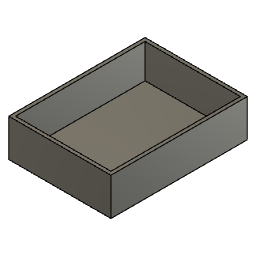
Box (Autodesk Fusion 360 design; units mm, degrees)
Autodesk Fusion 360 part; units mm, degrees
sketch "Sketch1" plane through (0, 0, 0) normal (0, 1, 0) x (1, 0, 0)
  line L0 (0, 0) -> (300, 0)
  line L1 (300, 0) -> (300, 400)
  line L2 (300, 400) -> (0, 400)
  line L3 (0, 400) -> (0, 0)
  line L4 (0, 0) -> (10, 0)
  line L5 (0, 0) -> (9.8603, 0)
  line L6 (0, 10) -> (0, 0)
  line L7 (9.8603, 10) -> (289.8603, 10)
  line L8 (289.8603, 10) -> (289.8603, 390)
  line L9 (289.8603, 390) -> (9.8603, 390)
  line L10 (9.8603, 390) -> (9.8603, 10)
  constraint horizontal L0
  constraint vertical L1
  constraint horizontal L2
  constraint vertical L3
  constraint coincident L0.start L3.end
  constraint perpendicular L3 L4
  constraint horizontal L5
  constraint vertical L6
  constraint horizontal L7
  constraint vertical L8
  constraint horizontal L9
  constraint vertical L10
extrude "Extrude1" add sketch "Sketch1" along normal blind 10 contours L0 L1 L2 L3 L4 L5 L6 | L7 L8 L9 L10
sketch "Sketch2" plane through (0, 10, 0) normal (0, 1, 0) x (-1, 0, 0)
  line L0 (0, -400) -> (0, 0)
  line L1 (0, 0) -> (-300, 0)
  line L2 (-300, 0) -> (-300, -400)
  line L3 (-300, -400) -> (0, -400)
  line L4 (0, 0) -> (-10, 0)
  line L5 (0, -10) -> (0, 0)
  line L6 (-10, -10) -> (-290, -10)
  line L7 (-290, -10) -> (-290, -390)
  line L8 (-290, -390) -> (-10, -390)
  line L9 (-10, -390) -> (-10, -10)
  line L10 (0, 0) -> (-300, 0)
  line L11 (-300, 0) -> (-300, -400)
  line L12 (-300, -400) -> (0, -400)
  line L13 (0, -400) -> (0, 0)
  constraint horizontal L4
  constraint vertical L5
  constraint coincident L0.end L1.start
  constraint horizontal L6
  constraint vertical L7
  constraint horizontal L8
  constraint vertical L9
  constraint horizontal L10
  constraint vertical L11
  constraint horizontal L12
  constraint vertical L13
  constraint coincident L2.end L3.start
extrude "Extrude2" add sketch "Sketch2" along normal blind 100
